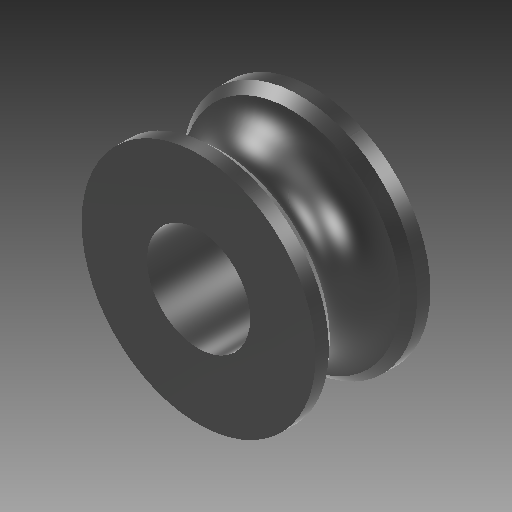
# Autodesk Inventor part: TTB 4mm Dyneema Cable Pulley
Saved by Autodesk Inventor 2023 (Build 270158000, 158)
## iProperties
Created: 2022-11-17
Part Number: TTB 4mm Dyneema Cable Pulley
Material: Acetal Resin, Black
Document SubType Name: Modeling
Designer: Max Boord
Mass: 7.28883 g
Surface Area: 30.9487 cm^2
Volume: 5.11497 cm^3
Density: 1.425 g/cm^3
Appearance: Satin - Black
Author: Max Boord
Autodesk Inventor part; units mm, degrees
ref_plane "YZ Plane" through (0, 0, 0) normal (1, 0, 0) x (0, 1, 0)
ref_plane "XZ Plane" through (0, 0, 0) normal (0, 1, 0) x (-1, 0, 0)
ref_plane "XY Plane" through (0, 0, 0) normal (0, 0, 1) x (1, 0, 0)
sketch "Sketch1" plane through (0, 0, 0) normal (0, 1, 0) x (-1, 0, 0)
  line L0 (-6.4389, 0) -> (-6.4389, -7.167)
  line L1 (-14.605, -5.5) -> (-13.605, -4.3875)
  line L2 (-14.605, -7.167) -> (-14.605, -5.5)
  line L3 (-6.4389, -7.167) -> (-14.605, -7.167)
  line L4 (-6.4389, 0) -> (-6.4389, -7.167)
  arc A0 (-13.605, -4.3875) -> (-10.105, 0) centre (-14.605, 0) ccw
  line L5 (0, 7.167) -> (0, -7.167)
  line L6 (-10.105, 0) -> (-6.4389, 0)
  point P0 (0, 0)
  point P1 (0, 0)
  dimension "d0" = 12.8778
  dimension "d1" = 29.21
  dimension "d2" = 1.667
  dimension "d3" = 4.5
  dimension "d6" = 8.1661
  dimension "d7" = 1
  dimension "d8" = 11
  constraints: 14 end point, 3 horizontal alignment, 2 centre point, 2 coincident, 2 point on circle, 1 horizontal, 1 midpoint, 1 perpendicular, 1 vertical
  measures "d0" diameter of L0 L5
  measures "d1" diameter of L2 L5
  measures "d2" distance of L2.start L1.start
  measures "d3" radius of A0
  measures "d6" distance from line of L0 A0.centre
  measures "d7" distance from line of L2 L1.end
  measures "d8" diameter of L1.start L6
revolve "Revolution1" add sketch "Sketch1" angle 360 about axis through (0, 0, 7.167) along (0, 0, -1)
mirror "Mirror1" about plane through (10.105, 0, 0) normal (0, 0, 1)
body "Solid1"
